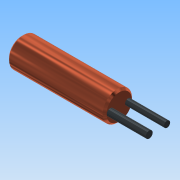
# Autodesk Inventor part: термодатчик1
Saved by Autodesk Inventor 2017 (Build 210142000, 142)
## iProperties
Part Number: термодатчик1
Material: Типовые
Document SubType Name: Modeling
Designer: Max
Mass: 0.0731543 g
Surface Area: 1.22899 cm^2
Volume: 0.0731543 cm^3
Density: 1 g/cm^3
Appearance: Металл — 1400F
Author: Max
Autodesk Inventor part; units mm, degrees
ref_plane "YZ Plane" through (0, 0, 0) normal (1, 0, 0) x (0, 1, 0)
ref_plane "XZ Plane" through (0, 0, 0) normal (0, 1, 0) x (-1, 0, 0)
ref_plane "XY Plane" through (0, 0, 0) normal (0, 0, 1) x (1, 0, 0)
sketch "Эскиз1" plane through (0, 0, 0) normal (1, 0, 0) x (0, 1, 0)
  circle A0 centre (0, 0) radius 1.5
  dimension "d0" = 3
  constraints: 1 centre point, 1 coincident
  measures "d0" diameter of A0
extrude "Выдавливание1" add sketch "Эскиз1" along normal blind 10
sketch "Эскиз2" plane through (10, 0, 0) normal (1, 0, 0) x (0, 0, -1)
  circle A0 centre (0, 0.9066) radius 0.3125
  circle A1 centre (0, -0.9266) radius 0.357
  point P0 (0, 0)
  constraints: 2 centre point
extrude "Выдавливание2" add sketch "Эскиз2" along normal blind 4
chamfer "Фаска1" distance 0.2 angle 45 2 edges at (10, -1.5, 0) (0, -1.5, 0)
